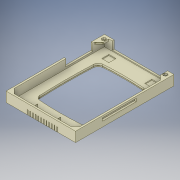
# Autodesk Inventor part: watch
Saved by Autodesk Inventor 2017 (Build 210142000, 142)
## iProperties
Created: 2018-03-02
Part Number: watch
Material: ABS Plastic
Document SubType Name: Modeling
Designer: Chad
Density: 1.06 g/cm^3
Appearance: Smooth - White
Author: Chad
Autodesk Inventor part; units mm, degrees
ref_plane "YZ Plane" through (0, 0, 0) normal (1, 0, 0) x (0, 1, 0)
ref_plane "XZ Plane" through (0, 0, 0) normal (0, 1, 0) x (-1, 0, 0)
ref_plane "XY Plane" through (0, 0, 0) normal (0, 0, 1) x (1, 0, 0)
sketch "Top Face" plane through (0, 0, 0) normal (0, 1, 0) x (-1, 0, 0)
  line L0 (-23.495, 34.925) -> (25.8445, 34.925)
  line L1 (25.8445, 34.925) -> (25.8445, -34.925)
  line L2 (25.8445, -34.925) -> (-23.495, -34.925)
  line L3 (-23.495, -34.925) -> (-23.495, 34.925)
  point P0 (0, 0)
  dimension "d0" = 69.85
  dimension "d107" = 25.8445
  dimension "d108" = 34.925
  dimension "d110" = 23.495
  constraints: 8 end point, 2 parallel, 1 horizontal, 1 perpendicular
  measures "d0" distance of L0.end L1.end
  measures "d107" horizontal distance of L1.end point (0, 0)
  measures "d108" vertical distance of point (0, 0) L0.end
  measures "d110" horizontal distance of L2.end point (0, 0)
extrude "Top Face Ext" add sketch "Top Face" along normal blind 7.62
shell "Shell2" thickness 1.27 removed faces 1 at (-9.398, 7.62, 11.6417)
sketch "Display" plane through (0, 0, 0) normal (0, -1, 0) x (1, 0, 0)
  line L0 (-18.053, 22.8672) -> (17.8373, -22.5939) construction
  line L1 (19.05, -24.13) -> (-19.05, -24.13)
  line L2 (-19.05, -24.13) -> (-19.05, 24.13)
  line L3 (-19.05, 24.13) -> (19.05, 24.13)
  line L4 (19.05, 24.13) -> (19.05, -24.13)
  line L5 (19.05, -24.13) -> (-19.05, 24.13) construction
  line L6 (-19.05, -24.13) -> (19.05, 24.13) construction
  arc A0 (17.3696, -22.0014) -> (17.3696, 22.0014) centre (-388.4345, 0) ccw
  arc A1 (-17.3696, -22.0014) -> (17.3696, -22.0014) centre (0, 180.4548) ccw
  arc A2 (-17.3696, 22.0014) -> (-17.3696, -22.0014) centre (388.4345, 0) ccw
  arc A3 (17.3696, 22.0014) -> (-17.3696, 22.0014) centre (0, -180.4548) ccw
  line L7 (-25.8445, 34.925) -> (-25.8445, -34.925) projected
  line L8 (23.495, 34.925) -> (-25.8445, 34.925) projected
  line L9 (23.495, -34.925) -> (23.495, 34.925) projected
  line L10 (-25.8445, -34.925) -> (23.495, -34.925) projected
  line L11 (19.5513, -24.765) -> (-19.5513, -24.765)
  line L12 (-19.5513, -24.765) -> (-19.5513, 24.765)
  line L13 (-19.5513, 24.765) -> (19.5513, 24.765)
  line L14 (19.5513, 24.765) -> (19.5513, -24.765)
  line L15 (19.5513, -24.765) -> (-19.5513, 24.765) construction
  line L16 (-19.5513, -24.765) -> (19.5513, 24.765) construction
  point P0 (0, 0)
  dimension "d35" = 38.1
  dimension "d36" = 48.26
  dimension "d37" = 203.2
  dimension "d38" = 203.2
  dimension "d39" = 406.4
  dimension "d40" = 406.4
  dimension "d41" = 22.0014
  dimension "d50" = 0.635
  constraints: 26 end point, 8 parallel, 8 point on circle, 7 point on line, 4 centre point, 4 midpoint, 2 horizontal, 2 horizontal alignment, 2 perpendicular, 2 vertical alignment
  measures "d35" distance of L1.start L1.end
  measures "d36" distance of L1.end L2.end
  measures "d37" radius of A1
  measures "d38" radius of A3
  measures "d39" radius of A0
  measures "d40" radius of A2
  measures "d41" vertical distance of A1.start point (0, 0)
  measures "d50" distance between parallel lines of L11 L1
sketch "Disp SD" plane through (23.495, 0, 34.925) normal (1, 0, 0) x (0, 0, -1)
  line L0 (43.053, 6.35) -> (19.05, 6.35)
  line L1 (19.05, 6.35) -> (19.05, 4.2418)
  line L2 (19.05, 4.2418) -> (43.053, 4.2418)
  line L3 (43.053, 4.2418) -> (43.053, 6.35)
  line L4 (69.85, 0) -> (0, 0) projected
  line L5 (0, 0) -> (0, 7.62) projected
  point P0 (34.925, 0)
  dimension "d19" = 2.1082
  dimension "d20" = 24.003
  dimension "d21" = 19.05
  dimension "d22" = 4.2418
  constraints: 8 end point, 2 parallel, 1 horizontal, 1 perpendicular
  measures "d19" distance of L0.end L1.end
  measures "d20" distance of L1.end L2.end
  measures "d21" distance between parallel lines of L5 L1
  measures "d22" distance from line of L4 L1.end
extrude "Disp SD Ext" cut sketch "Disp SD" against normal blind 5.08
extrude "Display Cut" cut sketch "Display" against normal blind 5.08 contours A1 A2 A3 A0
extrude "Display Rim" add sketch "Display" along normal blind 1.27 contours L1 L2 L3 L4
fillet "Disp Inner Fillet" radius 3.175 4 edges at (-17.3696, 0, -22.0014) (-17.3696, 0, 22.0014) (17.3696, 0, 22.0014) (17.3696, 0, -22.0014)
chamfer "Disp Inner Bevel" distance 0.635 distance2 1.27 8 edges at (-17.9655, -1.27, 0) (-16.6124, -1.27, 21.2729) (0, -1.27, 22.7452) (16.6124, -1.27, 21.2729) (17.9655, -1.27, 0) (16.6124, -1.27, -21.2729) (0, -1.27, -22.7452) (-16.6124, -1.27, -21.2729) measured on face at (1.6199, -1.27, -23.649)
extrude "Display Well" cut sketch "Display" against normal blind 0.635 contours L11 L12 L13 L14
sketch "Fans" plane through (0, 0, 0) normal (0, -1, 0) x (1, 0, 0)
  line L0 (-25.8445, 34.925) -> (23.495, 34.925) projected
  line L1 (10.16, 32.385) -> (10.795, 32.385)
  line L2 (10.795, 32.385) -> (10.795, 34.925)
  line L3 (10.795, 34.925) -> (10.16, 34.925)
  line L4 (10.16, 34.925) -> (10.16, 32.385)
  line L5 (22.225, 33.655) -> (-24.5745, 33.655) projected
  line L6 (10.16, 32.385) -> (10.795, 34.925) construction
  line L7 (10.795, 32.385) -> (10.16, 34.925) construction
  line L8 (23.495, 34.925) -> (-25.8445, 34.925) projected
  line L9 (23.495, -34.925) -> (23.495, 34.925) projected
  line L10 (8.255, 34.925) -> (8.255, 32.385)
  line L11 (8.89, 34.925) -> (8.255, 34.925)
  line L12 (8.89, 32.385) -> (8.89, 34.925)
  line L13 (8.255, 32.385) -> (8.89, 32.385)
  line L14 (6.35, 34.925) -> (6.35, 32.385)
  line L15 (6.985, 34.925) -> (6.35, 34.925)
  line L16 (6.985, 32.385) -> (6.985, 34.925)
  line L17 (6.35, 32.385) -> (6.985, 32.385)
  line L18 (4.445, 34.925) -> (4.445, 32.385)
  line L19 (5.08, 34.925) -> (4.445, 34.925)
  line L20 (5.08, 32.385) -> (5.08, 34.925)
  line L21 (4.445, 32.385) -> (5.08, 32.385)
  line L22 (2.54, 34.925) -> (2.54, 32.385)
  line L23 (3.175, 34.925) -> (2.54, 34.925)
  line L24 (3.175, 32.385) -> (3.175, 34.925)
  line L25 (2.54, 32.385) -> (3.175, 32.385)
  line L26 (0.635, 34.925) -> (0.635, 32.385)
  line L27 (1.27, 34.925) -> (0.635, 34.925)
  line L28 (1.27, 32.385) -> (1.27, 34.925)
  line L29 (0.635, 32.385) -> (1.27, 32.385)
  line L30 (-1.27, 34.925) -> (-1.27, 32.385)
  line L31 (-0.635, 34.925) -> (-1.27, 34.925)
  line L32 (-0.635, 32.385) -> (-0.635, 34.925)
  line L33 (-1.27, 32.385) -> (-0.635, 32.385)
  line L34 (-3.175, 34.925) -> (-3.175, 32.385)
  line L35 (-2.54, 34.925) -> (-3.175, 34.925)
  line L36 (-2.54, 32.385) -> (-2.54, 34.925)
  line L37 (-3.175, 32.385) -> (-2.54, 32.385)
  line L38 (-5.08, 34.925) -> (-5.08, 32.385)
  line L39 (-4.445, 34.925) -> (-5.08, 34.925)
  line L40 (-4.445, 32.385) -> (-4.445, 34.925)
  line L41 (-5.08, 32.385) -> (-4.445, 32.385)
  line L42 (-6.985, 34.925) -> (-6.985, 32.385)
  line L43 (-6.35, 34.925) -> (-6.985, 34.925)
  line L44 (-6.35, 32.385) -> (-6.35, 34.925)
  line L45 (-6.985, 32.385) -> (-6.35, 32.385)
  line L46 (-8.89, 34.925) -> (-8.89, 32.385)
  line L47 (-8.255, 34.925) -> (-8.89, 34.925)
  line L48 (-8.255, 32.385) -> (-8.255, 34.925)
  line L49 (-8.89, 32.385) -> (-8.255, 32.385)
  line L50 (-10.795, 34.925) -> (-10.795, 32.385)
  line L51 (-10.16, 34.925) -> (-10.795, 34.925)
  line L52 (-10.16, 32.385) -> (-10.16, 34.925)
  line L53 (-10.795, 32.385) -> (-10.16, 32.385)
  point P0 (0, 0)
  point P1 (10.4775, 33.655)
  dimension "d53" = 0.635
  dimension "d54" = 12.7
  dimension "d57" = 1.905
  constraints: 100 end point, 3 parallel, 2 horizontal, 2 midpoint, 2 point on line, 1 perpendicular, 88 other
  measures "d53" distance of L1.start L1.end
  measures "d54" distance between parallel lines of L9 L2
  measures "d57" distance of L3.end L10.start
extrude "Fans Cut" cut sketch "Fans" against normal blind 3.81 contours L0 L52 L5 L50 | L5 L52 L53 L50 | L0 L48 L5 L46 | L5 L48 L49 L46 | L0 L44 L5 L42 | L5 L44 L45 L42 | L0 L40 L5 L38 | L5 L40 L41 L38 | L0 L36 L5 L34 | L5 L36 L37 L34 | L0 L32 L5 L30 | L5 L32 L33 L30 | L0 L28 L5 L26 | L5 L28 L29 L26 | L0 L24 L5 L22 | L5 L24 L25 L22 | L0 L20 L5 L18 | L5 L20 L21 L18 | L0 L16 L5 L14 | L5 L16 L17 L14 | L0 L12 L5 L10 | L5 L12 L13 L10 | L0 L2 L5 L4 | L5 L2 L1 L4
chamfer "Outer bevel" distance 0.635 angle 45 16 edges at (17.145, 0, 34.925) (9.525, 0, 34.925) (7.62, 0, 34.925) (5.715, 0, 34.925) (3.81, 0, 34.925) (1.905, 0, 34.925) (0, 0, 34.925) (-1.905, 0, 34.925) (-3.81, 0, 34.925) (-5.715, 0, 34.925) (-7.62, 0, 34.925) (-9.525, 0, 34.925) (-18.3197, 0, 34.925) (23.495, 0, 0) (-1.1747, 0, -34.925) (-25.8445, 0, 0)
sketch "Logo" plane through (0, 0, 0) normal (0, -1, 0) x (1, 0, 0)
  line L0 (-19.5513, -25.4) -> (19.5513, -25.4)
  line L1 (19.5513, -25.4) -> (19.5513, -33.02)
  line L2 (19.5513, -33.02) -> (-19.5513, -33.02)
  line L3 (-19.5513, -33.02) -> (-19.5513, -25.4)
  line L4 (22.86, -34.29) -> (-25.2095, -34.29) projected
  line L5 (19.5513, 24.765) -> (19.5513, -24.765) projected
  line L6 (-19.5513, -24.765) -> (-19.5513, 24.765) projected
  arc A0 (-21.3312, -14.7974) -> (-21.3312, -16.9526) centre (-22.4088, -15.875) ccw construction
  arc A1 (-21.1516, -14.6178) -> (-21.1516, -17.1322) centre (-22.4088, -15.875) ccw
  arc A2 (-21.5108, -14.977) -> (-21.5108, -16.773) centre (-22.4088, -15.875) ccw
  arc A3 (-21.5108, -14.977) -> (-21.1516, -14.6178) centre (-21.3312, -14.7974) ccw
  arc A4 (-21.1516, -17.1322) -> (-21.5108, -16.773) centre (-21.3312, -16.9526) ccw
  line L7 (-25.8445, -34.925) -> (23.495, -34.925) projected
  line L8 (-21.9662, -15.875) -> (-20.6962, -15.875) construction
  line L9 (-21.9662, -15.621) -> (-20.6962, -15.621)
  line L10 (-20.6962, -16.129) -> (-21.9662, -16.129)
  arc A5 (-21.9662, -15.621) -> (-21.9662, -16.129) centre (-21.9662, -15.875) ccw
  arc A6 (-20.6962, -16.129) -> (-20.6962, -15.621) centre (-20.6962, -15.875) ccw
  point P0 (0, 0)
  point P1 (-21.3312, -15.875)
  dimension "d68" = 1.27
  dimension "d69" = 7.62
  dimension "d141" = 19.05
  dimension "d142" = 1.27
  dimension "d143" = 90
  dimension "d145" = 2.8575
  dimension "d147" = 0.508
  dimension "d149" = 0.508
  dimension "d150" = 1.27
  constraints: 16 end point, 14 point on circle, 8 tangent, 7 centre point, 3 parallel, 2 collinear, 2 horizontal, 2 vertical alignment, 1 horizontal alignment, 1 midpoint, 1 perpendicular
  measures "d68" distance between parallel lines of L4 L2
  measures "d69" distance of L2.end L0.start
  measures "d141" distance from line of L7 A0.centre
  measures "d142" radius of A2
  measures "d145" distance from line of L6 A0.centre
  measures "d147" distance between parallel lines of L9 L10
  measures "d149" radial gap between concentric circles of A1 A2
  measures "d150" distance of L9.start L9.end
extrude "Sticker Plate" cut sketch "Logo" against normal blind 0.254
sketch "Buttons" plane through (23.495, 7.62, -34.925) normal (0, 0, -1) x (-1, 0, 0)
  line L0 (1.27, 0) -> (48.0695, 0) projected
  line L1 (42.545, -5.715) -> (4.445, -5.715)
  line L2 (4.445, -5.715) -> (4.445, 0)
  line L3 (4.445, 0) -> (42.545, 0)
  line L4 (42.545, 0) -> (42.545, -5.715)
  line L5 (4.445, -8.89) -> (4.445, -6.985) projected
  line L6 (42.545, -6.985) -> (42.545, -8.89) projected
  line L7 (49.3395, -6.985) -> (0, -6.985) projected
  point P0 (23.495, -7.62)
  dimension "d72" = 1.27
  constraints: 8 end point, 2 collinear, 2 parallel, 1 horizontal, 1 perpendicular, 1 point on line
  measures "d72" distance between parallel lines of L7 L1
extrude "Button Cut" cut sketch "Buttons" against normal blind 1.27
sketch "PCB Supports" plane through (0, 7.62, 0) normal (0, 1, 0) x (1, 0, 0)
  line L0 (-10.795, -33.655) -> (-24.5745, -33.655) projected
  line L1 (-21.3995, -33.655) -> (-24.5745, -30.48)
  line L2 (-24.5745, -30.48) -> (-24.5745, -33.655)
  line L3 (-24.5745, -33.655) -> (-21.3995, -33.655)
  line L4 (-21.3995, -33.655) -> (-24.5745, -33.655)
  line L5 (22.225, 33.655) -> (22.225, -33.655) projected
  line L6 (22.225, -30.48) -> (19.05, -33.655)
  line L7 (22.225, -33.655) -> (10.795, -33.655) projected
  line L8 (22.225, -33.655) -> (19.05, -33.655)
  line L9 (22.225, -33.655) -> (22.225, -30.48)
  line L10 (-24.5745, -33.655) -> (-24.5745, 33.655) projected
  line L11 (19.05, 33.655) -> (22.225, 33.655)
  line L12 (22.225, 33.655) -> (22.225, 29.845)
  line L13 (22.225, 29.845) -> (19.05, 29.845)
  line L14 (19.05, 29.845) -> (19.05, 33.655)
  line L15 (-19.05, 33.655) -> (-19.05, 34.925) projected
  line L16 (19.05, 34.925) -> (19.05, 33.655) projected
  line L17 (19.05, 29.845) -> (22.225, 26.67)
  line L18 (22.225, 29.845) -> (22.225, 26.67)
  line L19 (-24.3491, 32.4832) -> (-23.0791, 33.2165)
  line L20 (-23.0791, 33.2165) -> (-21.8091, 32.4832)
  line L21 (-21.8091, 32.4832) -> (-21.8091, 31.0168)
  line L22 (-21.8091, 31.0168) -> (-23.0791, 30.2835)
  line L23 (-23.0791, 30.2835) -> (-24.3491, 31.0168)
  line L24 (-24.3491, 31.0168) -> (-24.3491, 32.4832)
  line L25 (19.2754, 32.4832) -> (20.5454, 33.2165)
  line L26 (20.5454, 33.2165) -> (21.8154, 32.4832)
  line L27 (21.8154, 32.4832) -> (21.8154, 31.0168)
  line L28 (21.8154, 31.0168) -> (20.5454, 30.2835)
  line L29 (20.5454, 30.2835) -> (19.2754, 31.0168)
  line L30 (19.2754, 31.0168) -> (19.2754, 32.4832)
  line L31 (-24.5745, 33.655) -> (-19.05, 33.655) projected
  line L32 (-24.5745, 33.655) -> (-21.3995, 33.655)
  line L33 (-21.3995, 33.655) -> (-21.3995, 29.845)
  line L34 (-21.3995, 29.845) -> (-24.5745, 29.845)
  line L35 (-24.5745, 29.845) -> (-24.5745, 33.655)
  line L36 (-21.3995, 29.845) -> (-24.5745, 26.67)
  line L37 (-24.5745, 29.845) -> (-24.5745, 26.67)
  line L38 (19.05, 33.655) -> (22.225, 33.655) projected
  point P0 (0, 0)
  point P1 (-24.5745, 24.3205)
  point P2 (-23.0791, 31.75)
  point P3 (20.5454, 31.75)
  dimension "d75" = 45
  dimension "d76" = 3.175
  dimension "d77" = 45
  dimension "d78" = 3.175
  dimension "d95" = 45
  dimension "d100" = 0.2254
  dimension "d101" = 1.27
  dimension "d102" = 1.27
  dimension "d103" = 1.905
  dimension "d104" = 0.2254
  dimension "d116" = 3.175
  dimension "d117" = 1.905
  dimension "d118" = 3.81
  dimension "d119" = 45
  constraints: 62 end point, 8 point on line, 7 collinear, 7 parallel, 4 perpendicular, 2 horizontal, 26 other
  measures "d75" angle of L0 L1
  measures "d76" distance of L1.end L0.end
  measures "d77" angle of L7 L6
  measures "d78" distance of L5.end L6.start
  measures "d95" angle of L13 L17
  measures "d100" distance between parallel lines of L10 L24
  measures "d101" distance from line of L21 point (-23.079, 31.75)
  measures "d102" distance from line of L27 point (20.545, 31.75)
  measures "d103" distance from line of L11 point (20.545, 31.75)
  measures "d104" distance between parallel lines of L14 L30
  measures "d116" distance between parallel lines of L35 L33
  measures "d117" vertical distance of L10.end point (-23.079, 31.75)
  measures "d118" distance between parallel lines of L31 L34
  measures "d119" angle of L34 L36
extrude "Extrusion18" add sketch "PCB Supports" against normal blind 1.27 contours L5 L13 L14 L11 | L10 L31 L33 L34
extrude "Nut Bank" cut sketch "PCB Supports" against normal blind 1.27 contours L19 L20 L21 L22 L23 L24 | L25 L26 L27 L28 L29 L30
extrude "Extrusion17" add sketch "PCB Supports" against normal blind 0.254 contours L0 L2 L1 | L5 L17 L13 | L5 L7 L6 | L10 L34 L36
sketch "Sketch13" plane through (-25.8445, 7.62, -34.925) normal (-1, 0, 0) x (0, 0, 1)
  line L0 (0, 0) -> (69.85, 0) projected
  line L1 (9.525, 0) -> (28.575, 0)
  line L2 (28.575, 0) -> (28.575, -5.08)
  line L3 (28.575, -5.08) -> (9.525, -5.08)
  line L4 (9.525, -5.08) -> (9.525, 0)
  line L5 (0, -6.985) -> (0, 0) projected
  point P0 (34.925, -7.62)
  dimension "d111" = 19.05
  dimension "d112" = 9.525
  dimension "d113" = 5.08
  constraints: 8 end point, 2 parallel, 1 horizontal, 1 perpendicular, 1 point on line
  measures "d111" distance between parallel lines of L4 L2
  measures "d112" distance between parallel lines of L5 L4
  measures "d113" distance of L3.end L1.start
extrude "Power Button Cutout" cut sketch "Sketch13" against normal blind 1.27
pattern_linear "Rectangular Pattern2" count 2 spacing 1.016 along (0, -1, 0) of "Extrusion17"
sketch "Disp Support Sketch" plane through (-24.5745, 1.27, -33.655) normal (0, 1, 0) x (1, 0, 0)
  line L0 (0, -8.255) -> (0, -6.985) projected
  line L1 (41.91, -3.175) -> (36.83, -3.175)
  line L2 (36.83, -3.175) -> (36.83, -8.255)
  line L3 (36.83, -8.255) -> (41.91, -8.255)
  line L4 (41.91, -8.255) -> (41.91, -3.175)
  line L5 (6.35, -3.175) -> (11.43, -3.175)
  line L6 (11.43, -3.175) -> (11.43, -8.255)
  line L7 (11.43, -8.255) -> (6.35, -8.255)
  line L8 (6.35, -8.255) -> (6.35, -3.175)
  line L9 (5.0232, -8.255) -> (44.1258, -8.255) projected
  line L10 (0, -67.31) -> (0, 0) projected
  point P0 (24.5745, -33.655)
  dimension "d156" = 0
  dimension "d157" = 5.08
  dimension "d158" = 25.4
  dimension "d159" = 6.35
  constraints: 16 end point, 4 parallel, 2 equal length, 2 horizontal, 2 perpendicular, 2 point on line
  measures "d156" distance between parallel lines of L9 L7
  measures "d157" distance between parallel lines of L3 L1
  measures "d158" distance between parallel lines of L6 L2
  measures "d159" distance between parallel lines of L10 L8
extrude "Display Support" cut sketch "Disp Support Sketch" against normal blind 0.635
sketch "Sketch16" plane through (-10.795, 1.27, 33.655) normal (0, 0, -1) x (-1, 0, 0)
  line L0 (-4.0005, 3.81) -> (-4.2545, 3.81)
  line L1 (-4.2545, 3.81) -> (-4.2545, 6.35)
  line L2 (-4.2545, 6.35) -> (-4.0005, 6.35)
  line L3 (-4.0005, 6.35) -> (-4.0005, 3.81)
  line L4 (15.0495, 6.35) -> (-34.29, 6.35) projected
  line L5 (-20.2545, 3.81) -> (-20.5085, 3.81)
  line L6 (-20.5085, 3.81) -> (-20.5085, 6.35)
  line L7 (-20.5085, 6.35) -> (-20.2545, 6.35)
  line L8 (-20.2545, 6.35) -> (-20.2545, 3.81)
  line L9 (-29.845, 6.35) -> (10.6045, 6.35) projected
  line L10 (13.7795, 0) -> (13.7795, 5.08) projected
  point P0 (-10.795, -1.27)
  dimension "d175" = 2.54
  dimension "d176" = 16
  dimension "d177" = 0.254
  dimension "d178" = 0.254
  dimension "d179" = 17.78
  constraints: 16 end point, 4 parallel, 2 horizontal, 2 perpendicular, 2 point on line, 1 collinear
  measures "d175" distance of L2.end L0.start
  measures "d176" distance of L7.end L1.end
  measures "d177" distance between parallel lines of L1 L3
  measures "d178" distance of L5.start L5.end
  measures "d179" distance between parallel lines of L10 L3
extrude "Extrusion20" add sketch "Sketch16" along normal blind 2
thicken "Thicken1" operation cut thickness 0.1 both sides no extend neighbours no toward (0.9993241, 0, -0.0367614) faces at (17.6908, 0.8467, -14.9398) (16.7859, 0.4233, 21.0799) (-11.3342, 0.4233, 22.4288) (16.7859, 0.8467, -21.0799) (-11.3342, 0.8467, -22.4288) (-16.4237, 0.8467, -21.4511) (-17.9599, 0.8467, 2.1347) (-16.7859, 0.8467, 21.0799)
equation "\"d107\" = 1.1 * d110"
equation "\"d108\" = 0.5 * d0"
equation "\"d38\" = d37"
equation "\"d40\" = d39"
equation "\"d141\" = d112 + 0.5 * d111"
equation "\"d147\" = d149"
equation "\"d150\" = d142"
equation "\"d77\" = d75"
equation "\"d78\" = d76"
equation "\"d95\" = d75"
equation "\"d102\" = d101"
equation "\"d103\" = d117"
equation "\"d104\" = d100"
equation "\"d116\" = d76"
equation "\"d118\" = 2 * d117"
equation "\"d119\" = d95"
equation "\"d99\" = 0.5 * d93"
equation "\"d93\" = 3.81"
body "Solid1"
